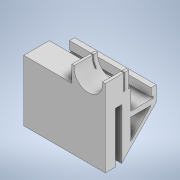
# Autodesk Inventor part: Base Part
Saved by Autodesk Inventor 2020 (Build 240168000, 168)
## iProperties
Created: 2020-11-24
Part Number: Base Part
Material: Generic
Document SubType Name: Modeling
Designer: shaun
Density: 1 g/cm^3
Appearance: Default
Author: shaun
Autodesk Inventor part; units mm, degrees
ref_plane "YZ Plane" through (0, 0, 0) normal (1, 0, 0) x (0, 1, 0)
ref_plane "XZ Plane" through (0, 0, 0) normal (0, 1, 0) x (-1, 0, 0)
ref_plane "XY Plane" through (0, 0, 0) normal (0, 0, 1) x (1, 0, 0)
sketch "Base" plane through (0, 0, 0) normal (1, 0, 0) x (0, 1, 0)
  line L0 (0, 0) -> (0, 6)
  line L1 (0, 6) -> (-50, 6)
  line L2 (-50, 6) -> (-50, 16)
  line L3 (-50, 16) -> (10, 16)
  line L4 (10, -9) -> (-10, -9)
  line L5 (-10, -9) -> (-10, -29)
  line L6 (-10, -29) -> (0, -29)
  line L7 (0, -29) -> (0, -34)
  line L8 (0, -34) -> (-15, -34)
  line L9 (-15, -34) -> (-50, 0)
  line L10 (-50, 0) -> (0, 0)
  line L11 (10, 16) -> (10, -9)
  dimension "d0" = 6
  dimension "d1" = 50
  dimension "d2" = 10
  dimension "d3" = 60
  dimension "d4" = 25
  dimension "d5" = 20
  dimension "d6" = 20
  dimension "d7" = 10
  dimension "d8" = 5
  dimension "d9" = 15
  constraints: 24 end point, 5 perpendicular, 3 point on line, 2 vertical, 1 parallel
  measures "d0" distance of L0.start L0.end
  measures "d1" distance of L0.end L1.end
  measures "d2" distance of L1.end L2.end
  measures "d3" distance of L2.end L3.end
  measures "d4" distance of L3.end L4.start
  measures "d5" distance of L4.start L4.end
  measures "d6" distance of L4.end L5.end
  measures "d7" distance of L5.end L6.end
  measures "d8" distance of L6.end L7.end
  measures "d9" distance of L7.end L8.end
sketch "Mount" plane through (0, 0, 0) normal (1, 0, 0) x (0, 1, 0)
  line L0 (10, 16) -> (26, 16)
  line L1 (26, 16) -> (26, -7)
  line L2 (26, -7) -> (10, -7)
  line L3 (10, -7) -> (10, 16)
  point P0 (0, 0)
  dimension "d13" = 16
  dimension "d14" = 23
  constraints: 8 end point, 3 perpendicular, 1 horizontal
  measures "d13" distance of L0.start L0.end
  measures "d14" distance of L0.end L1.end
extrude "Extrusion1" add sketch "Base" along normal blind 90
extrude "Extrusion2" add sketch "Mount" along normal blind 90
sketch "Sketch4" plane through (0, 10, -7) normal (0, 0, -1) x (-1, 0, 0)
  line L0 (0, 0) -> (0, 16) projected
  line L1 (0, 16) -> (-90, 16) projected
  line L2 (-90, 0) -> (-90, 16) projected
  line L3 (0, 0) -> (-90, 0) projected
  line L4 (-90, 17.3769) -> (-85, 17.3769)
  line L5 (-85, 17.3769) -> (-85, 0)
  line L6 (0, 0) -> (-90, 0) projected
  line L7 (-85, 0) -> (-62.2, 0)
  line L8 (-62.2, 0) -> (-62.2, 17.3769)
  line L9 (-62.2, 17.3769) -> (-57.2, 17.3769)
  line L10 (-57.2, 17.3769) -> (-57.2, 0)
  line L11 (-90, 17.3769) -> (-90, 25.7938)
  line L12 (-90, 25.7938) -> (16.0885, 26.6461)
  line L13 (16.0885, 26.6461) -> (17.0474, 0)
  line L14 (17.0474, 0) -> (-57.2, 0)
  point P0 (0, -10)
  dimension "d19" = 5
  dimension "d20" = 22.8
  dimension "d21" = 5
  constraints: 20 end point, 6 point on line, 3 perpendicular, 1 collinear, 1 horizontal, 1 vertical
  measures "d19" distance of L4.start L4.end
  measures "d20" distance of L5.end L7.end
  measures "d21" distance of L8.end L9.end
extrude "Extrusion3" cut sketch "Sketch4" against normal blind 90 contours L3 L10 L1 L0 | L0 L1 L10 L9 L8 L5 L4 L11 L12 L13 L14 | L3 L5 L1 L8
sketch "Sketch7" plane through (90, 0, 0) normal (1, 0, 0) x (0, 0, -1)
  line L0 (29, 0) -> (29, -10) projected
  line L1 (29, -10) -> (9, -10) projected
  line L2 (9, -10) -> (9, 10) projected
  line L3 (9, 10) -> (7, 10) projected
  line L4 (7, 10) -> (7, 26) projected
  line L5 (7, 26) -> (-16, 26) projected
  line L6 (-16, 26) -> (-16, -50) projected
  line L7 (-16, -50) -> (-6, -50) projected
  line L8 (-6, -50) -> (-6, 0) projected
  line L9 (-6, 0) -> (0, 0) projected
  line L10 (0, 0) -> (0, -50) projected
  line L11 (0, -50) -> (34, -15) projected
  line L12 (34, -15) -> (34, 0) projected
  line L13 (34, 0) -> (29, 0) projected
  line L14 (9, -15) -> (29, -15)
  line L15 (29, -15) -> (9, -35.6361)
  line L16 (9, -35.6361) -> (9, -15)
  constraints: 6 end point, 1 horizontal, 1 perpendicular
extrude "Extrusion5" cut sketch "Sketch7" against normal blind 90 contours L14 L15 L16
sketch "Sketch8" plane through (90, 0, 0) normal (1, 0, 0) x (0, 0, -1)
  line L0 (29, -15) -> (9, -35.6361) projected
  line L1 (9, -35.6361) -> (9, -15) projected
  line L2 (9, -15) -> (29, -15) projected
  line L3 (29, 0) -> (29, -10) projected
  line L4 (29, -10) -> (9, -10) projected
  line L5 (9, -10) -> (9, 10) projected
  line L6 (9, 10) -> (7, 10) projected
  line L7 (7, 10) -> (7, 26) projected
  line L8 (7, 26) -> (-16, 26) projected
  line L9 (-16, 26) -> (-16, -50) projected
  line L10 (-16, -50) -> (-6, -50) projected
  line L11 (-6, -50) -> (-6, 0) projected
  line L12 (-6, 0) -> (0, 0) projected
  line L13 (0, 0) -> (0, -50) projected
  line L14 (0, -50) -> (34, -15) projected
  line L15 (34, -15) -> (34, 0) projected
  line L16 (34, 0) -> (29, 0) projected
  line L17 (2, 10) -> (3, 10)
  line L18 (2, 10) -> (2, 28)
  line L19 (2, 28) -> (3, 28)
  line L20 (3, 28) -> (3, 10)
  point P0 (-16, 10)
  dimension "d39" = 18
  dimension "d40" = 1
  dimension "d69" = 18
  constraints: 8 end point, 1 perpendicular, 1 point on line, 1 vertical
  measures "d39" distance of point (-16, 10) L17.start
  measures "d40" distance of L17.start L17.end
  measures "d69" distance from line of L18.end L17
extrude "Extrusion6" cut sketch "Sketch8" against normal blind 90 contours L20 L17 L18 L8 | L8 L18 L19 L20
sketch "Sketch9" plane through (0, -15, -34) normal (0, 0, -1) x (-1, 0, 0)
  line L0 (0, -35) -> (-90, -35) projected
  line L1 (0, -35) -> (-10, -35)
  line L2 (-10, -35) -> (-10, 26.7876)
  line L3 (-10, 26.7876) -> (0, 26.7876)
  line L4 (0, 26.7876) -> (0, -35)
  point P0 (0, 15)
  dimension "d44" = 10
  constraints: 8 end point, 2 parallel, 1 horizontal, 1 perpendicular
  measures "d44" distance of L2.end L3.end
extrude "Extrusion7" cut sketch "Sketch9" against normal blind 90
sketch "Sketch10" plane through (90, -10, -9) normal (0, 1, 0) x (1, 0, 0)
  line L0 (-74.3662, 20.0264) -> (-66.3662, 20.0264)
  line L1 (-66.3662, 20.0264) -> (-66.3662, 0.0264)
  line L2 (-66.3662, 0.0264) -> (-74.3662, 0.0264)
  line L3 (-74.3662, 0.0264) -> (-74.3662, 20.0264)
  point P0 (-90, -9)
  dimension "d47" = 8
  dimension "d58" = 20
  constraints: 8 end point, 2 parallel, 1 horizontal, 1 perpendicular
  measures "d47" distance of L1.end L2.end
  measures "d58" distance between parallel lines of L0 L2
extrude "Extrusion8" cut sketch "Sketch10" against normal blind 90
sketch "Sketch11" plane through (90, -50, 6) normal (0, -1, 0) x (1, 0, 0)
  line L0 (-74.3662, -35.0264) -> (-74.3662, -15.0264) projected
  line L1 (-74.3662, -15.0264) -> (-66.3662, -15.0264) projected
  line L2 (-66.3662, -15.0264) -> (-66.3662, -35.0264) projected
  line L3 (-66.3662, -35.0264) -> (-74.3662, -35.0264) projected
  line L4 (-80, -6) -> (-80, -40) projected
  line L5 (-80, -40) -> (0, -40) projected
  line L6 (0, -6) -> (0, -40) projected
  line L7 (-80, -6) -> (0, -6) projected
  line L8 (-60.2122, -34.9767) -> (-76.9534, -34.9767)
  line L9 (-76.9534, -34.9767) -> (-76.9534, -15.0247)
  line L10 (-76.9534, -15.0247) -> (-60.2122, -15.0247)
  line L11 (-60.2122, -15.0247) -> (-60.2122, -34.9767)
  point P0 (-90, -6)
  constraints: 8 end point, 2 parallel, 1 horizontal, 1 perpendicular
extrude "Extrusion9" cut sketch "Sketch11" against normal blind 35 contours L8 L9 L10 L0 | L2 L10 L11 L8
sketch "Sketch12" plane through (90, 10, -7) normal (0, 0, -1) x (-1, 0, 0)
  line L0 (5, 0) -> (5, 16) projected
  line L1 (5, 16) -> (0, 16) projected
  line L2 (0, 0) -> (0, 16) projected
  line L3 (5, 0) -> (0, 0) projected
  line L4 (27.8, 16) -> (27.8, 0) projected
  line L5 (32.8, 0) -> (27.8, 0) projected
  line L6 (32.8, 0) -> (32.8, 16) projected
  line L7 (32.8, 16) -> (27.8, 16) projected
  line L8 (2.5, 7) -> (16.4, 7)
  line L9 (80, 0) -> (0, 0) projected
  point P0 (90, -10)
  point P1 (30.282, 6.0006)
  dimension "d52" = 27.8
  dimension "d53" = 13.9
  dimension "d70" = 7
  constraints: 2 end point, 1 coincident, 1 horizontal
  measures "d52" distance of point (30.282, 6.001) L8.start
  measures "d53" distance of L8.start L8.end
  measures "d70" distance from line of L9 L8.end
sketch "Sketch13" plane through (90, 0, 0) normal (1, 0, 0) x (0, 0, -1)
  line L0 (2, 10) -> (2, 26) projected
  line L1 (2, 26) -> (-16, 26) projected
  line L2 (-16, 26) -> (-16, -50) projected
  line L3 (-16, -50) -> (-6, -50) projected
  line L4 (-6, -50) -> (-6, 0) projected
  line L5 (-6, 0) -> (0, 0) projected
  line L6 (0, 0) -> (0, -50) projected
  line L7 (0, -50) -> (34, -15) projected
  line L8 (34, -15) -> (34, 0) projected
  line L9 (34, 0) -> (29, 0) projected
  line L10 (29, 0) -> (29, -10) projected
  line L11 (29, -10) -> (9, -10) projected
  line L12 (9, -10) -> (9, 10) projected
  line L13 (9, 10) -> (7, 10) projected
  line L14 (7, 10) -> (7, 26) projected
  line L15 (3, 26) -> (3, 10) projected
  line L16 (3, 10) -> (2, 10) projected
  line L17 (29, -15) -> (9, -35.6361) projected
  line L18 (9, -35.6361) -> (9, -15) projected
  line L19 (9, -15) -> (29, -15) projected
  line L20 (29, -10) -> (9, -10) projected
  line L21 (29, -10) -> (31, -10)
  line L22 (31, -10) -> (31, -8)
  line L23 (31, -8) -> (29, -8)
  line L24 (29, 0) -> (29, -10) projected
  line L25 (29, -10) -> (29, -8)
  line L26 (7, 26) -> (3, 26) projected
  dimension "d54" = 2
  dimension "d55" = 2
  constraints: 8 end point, 2 perpendicular, 1 collinear, 1 horizontal, 1 point on line
  measures "d54" distance of L10.end L21.end
  measures "d55" distance of L21.end L22.end
extrude "Extrusion10" cut sketch "Sketch13" against normal through all contours L10 L23 L22 L21
sketch "Sketch15" plane through (90, 10, -7) normal (0, 0, -1) x (-1, 0, 0)
  line L0 (5, 0) -> (5, 16) projected
  line L1 (5, 16) -> (0, 16) projected
  line L2 (0, 0) -> (0, 16) projected
  line L3 (5, 0) -> (0, 0) projected
  line L4 (27.8, 16) -> (27.8, 0) projected
  line L5 (32.8, 0) -> (27.8, 0) projected
  line L6 (32.8, 0) -> (32.8, 16) projected
  line L7 (32.8, 16) -> (27.8, 16) projected
  line L8 (80, 0) -> (0, 0) projected
  circle A0 centre (16.6079, 14) radius 14 construction
  line L9 (27.8, 0) -> (27.8, 16) projected
  line L10 (27.8, 5.5895) -> (27.8, 16)
  line L11 (27.8, 16) -> (30.4643, 16)
  line L12 (32.8, 16) -> (27.8, 16) projected
  arc A1 (27.8, 5.5895) -> (30.4643, 16) centre (16.6079, 14) ccw
  line L13 (5, 16) -> (0, 16) projected
  line L14 (5, 16) -> (5, 0) projected
  arc A2 (2.7515, 16) -> (5, 6.1733) centre (16.6079, 14) ccw
  line L15 (5, 16) -> (2.7515, 16)
  line L16 (5, 6.1733) -> (5, 16)
  point P0 (90, -10)
  point P1 (27.8, 5.5895)
  point P2 (30.4643, 16)
  point P3 (2.7515, 16)
  point P4 (5, 6.1733)
  dimension "d63" = 14
  dimension "d64" = 28
  constraints: 8 end point, 8 point on circle, 4 point on line, 3 centre point, 2 concentric, 1 coincident, 1 collinear, 1 horizontal, 1 perpendicular
  measures "d63" distance from line of L8 point (16.608, 14)
  measures "d64" diameter of A0
extrude "Extrusion12" cut sketch "Sketch15" against normal up to surface (23 mm away) contours A2 L1 L0 | L4 L7 A1
sketch "Sketch16" plane through (90, 10, -7) normal (0, 0, -1) x (-1, 0, 0)
  circle A0 centre (16.6079, 14) radius 14 construction
  line L0 (5, 0) -> (5, 6.1733) projected
  line L1 (5, 6.1733) -> (5, 0)
  line L2 (5, 0) -> (27.7766, 0)
  line L3 (80, 0) -> (0, 0) projected
  line L4 (27.8, 0) -> (27.8, 5.5895) projected
  line L5 (27.8, 5.5895) -> (27.8, 0)
  line L6 (5, 0) -> (0, 0) projected
  line L7 (27.8, 0) -> (5, 0)
  line L8 (5, 0) -> (5, 6.1733)
  line L9 (32.8, 0) -> (27.8, 0) projected
  line L10 (5, 0) -> (27.8, 0)
  arc A1 (5, 6.1733) -> (27.8, 5.5895) centre (16.6079, 14) ccw
  point P0 (90, -10)
  point P1 (16.6079, 0)
  constraints: 12 end point, 2 collinear, 2 perpendicular, 2 point on circle, 1 centre point, 1 horizontal, 1 point on line
extrude "Extrusion13" add sketch "Sketch16" against normal up to surface (23 mm away)
body "Solid1"
